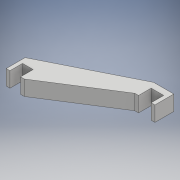
# Autodesk Inventor part: StrumArm
Saved by Autodesk Inventor 2017 (Build 210142000, 142)
## iProperties
Created: 2017-12-03
Part Number: StrumArm
Material: Generic
Document SubType Name: Modeling
Designer: Max
Density: 1 g/cm^3
Appearance: Default
Author: Max
Autodesk Inventor part; units mm, degrees
ref_plane "YZ Plane" through (0, 0, 0) normal (1, 0, 0) x (0, 1, 0)
ref_plane "XZ Plane" through (0, 0, 0) normal (0, 1, 0) x (-1, 0, 0)
ref_plane "XY Plane" through (0, 0, 0) normal (0, 0, 1) x (1, 0, 0)
sketch "Sketch1" plane through (0, 0, 0) normal (0, 0, 1) x (1, 0, 0)
  line L0 (0, 0) -> (0, 5)
  line L1 (0, 5) -> (4.2, 5)
  line L2 (4.2, 5) -> (4.2, 0)
  line L3 (4.2, 0) -> (5.7, 0)
  line L4 (-1.5, 7.5) -> (-1.5, 0)
  line L5 (-1.5, 0) -> (0, 0)
  line L6 (40.5, 24.5) -> (40.5, 17)
  line L7 (40.5, 17) -> (39, 17)
  line L8 (39, 17) -> (39, 22)
  line L9 (39, 22) -> (34, 22)
  line L10 (34, 22) -> (34, 17)
  line L11 (34, 17) -> (32.5, 17)
  line L12 (40.5, 24.5) -> (32.5, 24.5)
  line L13 (32.5, 17) -> (32.5, 24.5)
  line L14 (-1.5, 7.5) -> (5.7, 7.5)
  line L15 (5.7, 0) -> (5.7, 7.5)
  line L16 (-1.5, 7.5) -> (32.5, 24.5)
  line L17 (5.7, 0) -> (32.5, 17)
  dimension "d0" = 17
  dimension "d1" = 5
  dimension "d2" = 4.2
  dimension "d4" = 1.5
  dimension "d5" = 1.5
  dimension "d7" = 5
  dimension "d8" = 5
  dimension "d9" = 2.5
  dimension "d10" = 2.5
  dimension "d11" = 34
  constraints: 36 end point, 8 perpendicular, 4 vertical, 3 point on line, 2 collinear, 2 horizontal
  measures "d0" distance between parallel lines of L9 L1
  measures "d1" distance of L8.end L9.end
  measures "d2" distance of L0.end L1.end
  measures "d4" distance of L4.end L0.start
  measures "d5" distance of L10.end L11.end
  measures "d7" distance of L9.end L10.end
  measures "d8" distance of L1.end L2.end
  measures "d9" distance between parallel lines of L12 L9
  measures "d10" distance between parallel lines of L14 L1
  measures "d11" distance between parallel lines of L10 L0
extrude "Extrusion1" add sketch "Sketch1" along normal blind 6
body "Solid1"
